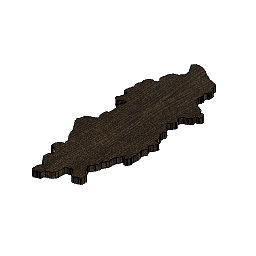
model (Autodesk Fusion 360 design; units mm, degrees)
Autodesk Fusion 360 part; units mm, degrees
(part 1 of 2)
sketch "Sketch1" plane through (0, 0, 0) normal (0, 0, 1) x (1, 0, 0)
  spline S0 degree 3 poles (85.9896, 120.8052) (84.9842, 121.2285) (83.9523, 120.9375) (82.9998, 120.8052) knots 0 0 0 0 1 1 1 1
  spline S1 degree 3 poles (82.9998, 120.8052) (82.0738, 120.6994) (81.4123, 120.911) (80.8038, 121.4667) knots 0 0 0 0 1 1 1 1
  spline S2 degree 3 poles (80.8038, 121.4667) (80.645, 121.6254) (80.4863, 121.89) (80.4863, 122.1017) knots 0 0 0 0 1 1 1 1
  spline S3 degree 3 poles (80.4863, 122.1017) (80.5127, 122.7102) (80.5921, 123.3187) (80.645, 123.9273) knots 0 0 0 0 1 1 1 1
  spline S4 degree 3 poles (80.645, 123.9273) (80.645, 123.9802) (80.6715, 124.0331) (80.6979, 124.086) knots 0 0 0 0 1 1 1 1
  spline S5 degree 3 poles (80.6979, 124.086) (80.989, 124.6681) (81.1742, 125.356) (79.9042, 127.605) knots 0 0 0 0 1 1 1 1
  spline S6 degree 2 poles (79.9042, 127.605) (79.9042, 127.6315) (79.8777, 127.6579) knots 0 0 0 1 1 1
  spline S7 degree 3 poles (79.8777, 127.6579) (79.7719, 127.9225) (79.6925, 128.1606) (79.5867, 128.4252) knots 0 0 0 0 1 1 1 1
  spline S8 degree 3 poles (79.5867, 128.4252) (79.0575, 129.6158) (78.6077, 130.8594) (77.4435, 131.6796) knots 0 0 0 0 1 1 1 1
  spline S9 degree 3 poles (77.4435, 131.6796) (77.0731, 131.9442) (76.835, 132.4998) (76.7556, 132.976) knots 0 0 0 0 1 1 1 1
  spline S10 degree 3 poles (76.7556, 132.976) (76.6763, 133.4523) (76.8615, 133.9814) (76.9408, 134.4577) knots 0 0 0 0 1 1 1 1
  spline S11 degree 3 poles (76.9408, 134.4577) (77.0996, 135.516) (77.1525, 136.6008) (77.6817, 137.5798) knots 0 0 0 0 1 1 1 1
  spline S12 degree 3 poles (77.6817, 137.5798) (78.105, 138.3735) (77.8669, 139.3789) (77.0996, 139.8817) knots 0 0 0 0 1 1 1 1
  spline S13 degree 3 poles (77.0996, 139.8817) (76.6498, 140.1992) (76.4381, 140.596) (76.4381, 141.1781) knots 0 0 0 0 1 1 1 1
  spline S14 degree 3 poles (76.4381, 141.1781) (76.4381, 141.6544) (76.2529, 141.9983) (75.7502, 142.21) knots 0 0 0 0 1 1 1 1
  spline S15 degree 3 poles (75.7502, 142.21) (75.0887, 142.4746) (74.5596, 142.9508) (74.2156, 143.6123) knots 0 0 0 0 1 1 1 1
  spline S16 degree 3 poles (74.2156, 143.6123) (74.0833, 143.8769) (73.7658, 144.0621) (73.5012, 144.2208) knots 0 0 0 0 1 1 1 1
  spline S17 degree 3 poles (73.5012, 144.2208) (72.3371, 144.9352) (70.9612, 145.3585) (70.3792, 146.7608) knots 0 0 0 0 1 1 1 1
  spline S18 degree 3 poles (70.3792, 146.7608) (70.141, 147.3429) (69.9029, 147.925) (69.7177, 148.5071) knots 0 0 0 0 1 1 1 1
  spline S19 degree 3 poles (69.7177, 148.5071) (69.215, 149.9623) (69.506, 150.9148) (70.7231, 151.8673) knots 0 0 0 0 1 1 1 1
  spline S20 degree 3 poles (70.7231, 151.8673) (71.3581, 152.37) (72.046, 152.8198) (72.1519, 153.7194) knots 0 0 0 0 1 1 1 1
  spline S21 degree 3 poles (72.1519, 153.7194) (72.2577, 154.6719) (72.7604, 155.4656) (73.369, 156.2064) knots 0 0 0 0 1 1 1 1
  spline S22 degree 3 poles (73.369, 156.2064) (73.5277, 156.4181) (73.6865, 156.6298) (73.7923, 156.8679) knots 0 0 0 0 1 1 1 1
  spline S23 degree 3 poles (73.7923, 156.8679) (73.8717, 157.0002) (73.951, 157.1854) (73.8981, 157.3177) knots 0 0 0 0 1 1 1 1
  spline S24 degree 3 poles (73.8981, 157.3177) (73.5806, 158.5348) (73.4748, 159.8312) (72.3106, 160.6779) knots 0 0 0 0 1 1 1 1
  spline S25 degree 3 poles (72.3106, 160.6779) (71.3317, 161.3923) (70.5644, 162.2919) (70.2469, 163.5354) knots 0 0 0 0 1 1 1 1
  spline S26 degree 3 poles (70.2469, 163.5354) (70.194, 163.7206) (70.141, 163.9323) (70.1675, 164.1175) knots 0 0 0 0 1 1 1 1
  spline S27 degree 3 poles (70.1675, 164.1175) (70.4056, 165.6785) (71.2523, 166.9221) (72.6017, 167.6894) knots 0 0 0 0 1 1 1 1
  spline S28 degree 3 poles (72.6017, 167.6894) (73.8981, 168.4302) (75.274, 169.0387) (76.5969, 169.7531) knots 0 0 0 0 1 1 1 1
  spline S29 degree 3 poles (76.5969, 169.7531) (76.8879, 169.9119) (77.2054, 170.1235) (77.3377, 170.3881) knots 0 0 0 0 1 1 1 1
  spline S30 degree 3 poles (77.3377, 170.3881) (77.6552, 171.1289) (78.1579, 171.6581) (78.8458, 172.0814) knots 0 0 0 0 1 1 1 1
  spline S31 degree 3 poles (78.8458, 172.0814) (79.3221, 172.3725) (79.9835, 172.6635) (80.1688, 173.1133) knots 0 0 0 0 1 1 1 1
  spline S32 degree 3 poles (80.1688, 173.1133) (80.5127, 173.9071) (80.8831, 174.8067) (80.1423, 175.6533) knots 0 0 0 0 1 1 1 1
  spline S33 degree 3 poles (80.1423, 175.6533) (79.4015, 176.5) (79.9306, 177.0556) (80.8302, 177.2937) knots 0 0 0 0 1 1 1 1
  spline S34 degree 3 poles (80.8302, 177.2937) (81.5181, 177.4789) (82.2325, 177.5583) (82.894, 177.7964) knots 0 0 0 0 1 1 1 1
  spline S35 degree 3 poles (82.894, 177.7964) (83.3967, 177.9817) (84.0052, 178.2198) (84.2169, 178.6431) knots 0 0 0 0 1 1 1 1
  spline S36 degree 3 poles (84.2169, 178.6431) (84.6667, 179.5162) (84.9842, 180.4687) (85.1958, 181.4477) knots 0 0 0 0 1 1 1 1
  spline S37 degree 3 poles (85.1958, 181.4477) (85.3017, 182.0033) (85.2223, 182.6912) (84.9577, 183.1939) knots 0 0 0 0 1 1 1 1
  spline S38 degree 3 poles (84.9577, 183.1939) (84.6931, 183.7231) (84.164, 184.12) (83.6877, 184.4904) knots 0 0 0 0 1 1 1 1
  spline S39 degree 3 poles (83.6877, 184.4904) (83.2644, 184.8079) (82.7617, 185.046) (82.259, 185.2312) knots 0 0 0 0 1 1 1 1
  spline S40 degree 3 poles (82.259, 185.2312) (81.1742, 185.6017) (80.1423, 185.1519) (79.084, 184.9667) knots 0 0 0 0 1 1 1 1
  spline S41 degree 3 poles (79.084, 184.9667) (78.8988, 184.9402) (78.6606, 184.8608) (78.5019, 184.9402) knots 0 0 0 0 1 1 1 1
  spline S42 degree 3 poles (78.5019, 184.9402) (78.2108, 185.0196) (77.814, 185.5752) (77.5758, 186.0779) knots 0 0 0 0 1 1 1 1
  spline S43 degree 3 poles (77.5758, 186.0779) (77.5494, 186.1308) (77.5494, 186.1573) (77.5229, 186.2102) knots 0 0 0 0 1 1 1 1
  spline S44 degree 3 poles (77.5229, 186.2102) (77.47, 186.4483) (77.4171, 186.66) (77.3377, 186.8452) knots 0 0 0 0 1 1 1 1
  spline S45 degree 3 poles (77.3377, 186.8452) (75.7502, 190.0996) (73.9246, 188.4856) (67.7598, 191.7135) knots 0 0 0 0 1 1 1 1
  spline S46 degree 3 poles (67.7598, 191.7135) (64.77, 193.2746) (62.7856, 195.5235) (61.5421, 197.4285) knots 0 0 0 0 1 1 1 1
  spline S47 degree 3 poles (61.5421, 197.4285) (61.5156, 197.455) (61.5156, 197.4814) (61.4892, 197.5344) knots 0 0 0 0 1 1 1 1
  spline S48 degree 3 poles (61.4892, 197.5344) (61.4098, 197.746) (61.3304, 197.9312) (61.251, 198.1429) knots 0 0 0 0 1 1 1 1
  spline S49 degree 3 poles (61.251, 198.1429) (61.1717, 198.3017) (61.1188, 198.4604) (60.9865, 198.5133) knots 0 0 0 0 1 1 1 1
  spline S50 degree 3 poles (60.9865, 198.5133) (60.9071, 198.5662) (60.8013, 198.6191) (60.7483, 198.725) knots 0 0 0 0 1 1 1 1
  spline S51 degree 2 poles (60.7483, 198.725) (60.0075, 200.1008) (59.7165, 201.0533) knots 0 0 0 1 1 1
  line L0 (59.7165, 201.0533) -> (59.69, 201.2385)
  spline S52 degree 3 poles (59.69, 201.2385) (59.6106, 202.0852) (60.0869, 202.6408) (60.6954, 203.1964) knots 0 0 0 0 1 1 1 1
  spline S53 degree 3 poles (60.6954, 203.1964) (60.8277, 203.3287) (60.8806, 203.6462) (60.8542, 203.8844) knots 0 0 0 0 1 1 1 1
  spline S54 degree 3 poles (60.8542, 203.8844) (60.8013, 204.3871) (60.5102, 204.7046) (60.034, 204.9162) knots 0 0 0 0 1 1 1 1
  spline S55 degree 3 poles (60.034, 204.9162) (59.9546, 204.9427) (59.8752, 204.9956) (59.7958, 205.0485) knots 0 0 0 0 1 1 1 1
  spline S56 degree 3 poles (59.7958, 205.0485) (59.5313, 205.2073) (59.4783, 205.5777) (59.69, 205.8158) knots 0 0 0 0 1 1 1 1
  spline S57 degree 3 poles (59.69, 205.8158) (59.9546, 206.1069) (60.1927, 206.2391) (60.5631, 206.2656) knots 0 0 0 0 1 1 1 1
  spline S58 degree 3 poles (60.5631, 206.2656) (60.8806, 206.2921) (61.0923, 206.636) (60.96, 206.9271) knots 0 0 0 0 1 1 1 1
  spline S59 degree 3 poles (60.96, 206.9271) (60.6161, 207.7473) (60.0604, 208.4087) (59.5048, 209.0966) knots 0 0 0 0 1 1 1 1
  spline S60 degree 3 poles (59.5048, 209.0966) (58.3936, 210.4989) (58.6846, 212.2981) (60.1927, 213.0919) knots 0 0 0 0 1 1 1 1
  spline S61 degree 3 poles (60.1927, 213.0919) (60.6161, 213.3035) (61.1188, 213.33) (61.6479, 213.3829) knots 0 0 0 0 1 1 1 1
  spline S62 degree 3 poles (61.6479, 213.3829) (61.939, 213.4094) (62.1771, 213.7004) (62.0977, 213.9914) knots 0 0 0 0 1 1 1 1
  spline S63 degree 3 poles (62.0977, 213.9914) (61.939, 214.5206) (61.7273, 215.0762) (61.5421, 215.6054) knots 0 0 0 0 1 1 1 1
  spline S64 degree 3 poles (61.5421, 215.6054) (61.5421, 215.6319) (61.5156, 215.6583) (61.5156, 215.6848) knots 0 0 0 0 1 1 1 1
  spline S65 degree 3 poles (61.5156, 215.6848) (61.1717, 216.2669) (61.0923, 216.9019) (61.2246, 217.5898) knots 0 0 0 0 1 1 1 1
  spline S66 degree 3 poles (61.2246, 217.5898) (61.3569, 218.2512) (61.3569, 218.9127) (61.3833, 219.5741) knots 0 0 0 0 1 1 1 1
  spline S67 degree 3 poles (61.3833, 219.5741) (61.4098, 220.1033) (61.0923, 220.3944) (60.6425, 220.5266) knots 0 0 0 0 1 1 1 1
  spline S68 degree 3 poles (60.6425, 220.5266) (60.4044, 220.606) (60.1398, 220.6589) (59.8752, 220.7119) knots 0 0 0 0 1 1 1 1
  spline S69 degree 3 poles (59.8752, 220.7119) (58.7904, 220.95) (58.129, 221.9554) (58.1819, 223.0402) knots 0 0 0 0 1 1 1 1
  spline S70 degree 3 poles (58.1819, 223.0402) (58.2083, 223.5164) (58.0496, 223.8869) (57.6527, 224.2308) knots 0 0 0 0 1 1 1 1
  spline S71 degree 3 poles (57.6527, 224.2308) (56.8325, 224.9981) (56.6473, 226.03) (57.1236, 227.0619) knots 0 0 0 0 1 1 1 1
  spline S72 degree 3 poles (57.1236, 227.0619) (57.1765, 227.1677) (57.2029, 227.3264) (57.15, 227.3794) knots 0 0 0 0 1 1 1 1
  spline S73 degree 3 poles (57.15, 227.3794) (56.8061, 227.8821) (56.6208, 228.57) (55.8271, 228.6758) knots 0 0 0 0 1 1 1 1
  spline S74 degree 3 poles (55.8271, 228.6758) (44.9792, 230.2369) (37.2798, 234.3908) (34.2371, 236.5604) knots 0 0 0 0 1 1 1 1
  spline S75 degree 3 poles (34.2371, 236.5604) (34.2106, 236.5604) (34.2106, 236.5869) (34.1842, 236.5869) knots 0 0 0 0 1 1 1 1
  spline S76 degree 3 poles (34.1842, 236.5869) (34.1313, 236.6398) (34.0783, 236.6927) (34.0254, 236.7456) knots 0 0 0 0 1 1 1 1
  spline S77 degree 3 poles (34.0254, 236.7456) (33.999, 236.7721) (33.9725, 236.7985) (33.946, 236.7985) knots 0 0 0 0 1 1 1 1
  spline S78 degree 3 poles (33.946, 236.7985) (33.8931, 236.825) (33.8402, 236.8779) (33.7608, 236.9044) knots 0 0 0 0 1 1 1 1
  spline S79 degree 3 poles (33.7608, 236.9044) (33.7344, 236.9044) (33.7344, 236.9308) (33.7079, 236.9308) knots 0 0 0 0 1 1 1 1
  spline S80 degree 3 poles (33.7079, 236.9308) (31.1679, 238.8623) (26.5906, 239.7619) (26.1144, 239.8413) knots 0 0 0 0 1 1 1 1
  spline S81 degree 3 poles (26.1144, 239.8413) (26.0879, 239.8413) (26.0615, 239.8413) (26.035, 239.8413) knots 0 0 0 0 1 1 1 1
  spline S82 degree 3 poles (26.035, 239.8413) (25.0296, 239.8942) (24.0242, 239.9206) (23.0188, 239.9735) knots 0 0 0 0 1 1 1 1
  spline S83 degree 3 poles (23.0188, 239.9735) (22.8865, 239.9735) (22.7542, 240) (22.6219, 240) knots 0 0 0 0 1 1 1 1
  spline S84 degree 3 poles (22.6219, 240) (22.569, 240) (22.5425, 240) (22.4896, 240) knots 0 0 0 0 1 1 1 1
  spline S85 degree 3 poles (22.4896, 240) (21.5371, 239.8148) (20.5846, 239.656) (19.6321, 239.4708) knots 0 0 0 0 1 1 1 1
  spline S86 degree 3 poles (19.6321, 239.4708) (19.5792, 239.4444) (19.4998, 239.4179) (19.4469, 239.3915) knots 0 0 0 0 1 1 1 1
  spline S87 degree 3 poles (19.4469, 239.3915) (19.394, 239.365) (19.3675, 239.3385) (19.341, 239.3121) knots 0 0 0 0 1 1 1 1
  line L1 (19.341, 239.3121) -> (19.2087, 239.1798)
  spline S88 degree 3 poles (19.2087, 239.1798) (19.1823, 239.1533) (19.1558, 239.1269) (19.1029, 239.1004) knots 0 0 0 0 1 1 1 1
  spline S89 degree 3 poles (19.1029, 239.1004) (18.7854, 238.9417) (18.4944, 238.8094) (18.2033, 238.6506) knots 0 0 0 0 1 1 1 1
  line L2 (18.2033, 238.6506) -> (18.0446, 238.5448)
  spline S90 degree 3 poles (18.0446, 238.5448) (17.9917, 238.4919) (17.9388, 238.439) (17.8858, 238.3596) knots 0 0 0 0 1 1 1 1
  spline S91 degree 3 poles (17.8858, 238.3596) (17.8594, 238.3331) (17.8594, 238.2802) (17.8329, 238.2538) knots 0 0 0 0 1 1 1 1
  spline S92 degree 3 poles (17.8329, 238.2538) (16.9333, 237.5658) (16.2719, 236.7192) (15.875, 235.6608) knots 0 0 0 0 1 1 1 1
  spline S93 degree 3 poles (15.875, 235.6608) (15.8221, 235.5285) (15.8485, 235.3698) (15.9279, 235.2375) knots 0 0 0 0 1 1 1 1
  spline S94 degree 3 poles (15.9279, 235.2375) (16.0073, 235.1052) (16.1131, 234.9465) (16.1925, 234.8142) knots 0 0 0 0 1 1 1 1
  spline S95 degree 3 poles (16.1925, 234.8142) (16.4306, 234.4967) (16.6688, 234.1792) (16.9333, 233.8352) knots 0 0 0 0 1 1 1 1
  spline S96 degree 3 poles (16.9333, 233.8352) (18.6002, 231.4275) (20.2406, 228.9669) (21.934, 226.5856) knots 0 0 0 0 1 1 1 1
  spline S97 degree 3 poles (21.934, 226.5856) (22.4102, 225.9242) (22.516, 225.2098) (22.6483, 224.4954) knots 0 0 0 0 1 1 1 1
  spline S98 degree 3 poles (22.6483, 224.4954) (22.8335, 223.3312) (22.9923, 222.1671) (23.151, 221.0029) knots 0 0 0 0 1 1 1 1
  spline S99 degree 3 poles (23.151, 221.0029) (23.204, 220.606) (23.1246, 220.2092) (22.9129, 219.8652) knots 0 0 0 0 1 1 1 1
  spline S100 degree 3 poles (22.9129, 219.8652) (22.5954, 219.3096) (22.2515, 218.7804) (21.881, 218.2512) knots 0 0 0 0 1 1 1 1
  spline S101 degree 3 poles (21.881, 218.2512) (21.7488, 218.066) (21.5635, 217.8808) (21.3519, 217.775) knots 0 0 0 0 1 1 1 1
  spline S102 degree 3 poles (21.3519, 217.775) (20.664, 217.4575) (20.3465, 216.8754) (20.1083, 216.214) knots 0 0 0 0 1 1 1 1
  spline S103 degree 3 poles (20.1083, 216.214) (19.8967, 215.579) (19.5263, 215.1027) (18.8648, 214.8117) knots 0 0 0 0 1 1 1 1
  spline S104 degree 3 poles (18.8648, 214.8117) (17.3302, 214.0973) (15.7956, 213.33) (14.2875, 212.5362) knots 0 0 0 0 1 1 1 1
  spline S105 degree 3 poles (14.2875, 212.5362) (13.1763, 211.9277) (12.5148, 210.8429) (12.0915, 209.7052) knots 0 0 0 0 1 1 1 1
  spline S106 degree 3 poles (12.0915, 209.7052) (11.6417, 208.4881) (11.4565, 207.1917) (11.0331, 205.9746) knots 0 0 0 0 1 1 1 1
  spline S107 degree 3 poles (11.0331, 205.9746) (11.0067, 205.8687) (10.9538, 205.7894) (10.9273, 205.6835) knots 0 0 0 0 1 1 1 1
  spline S108 degree 3 poles (10.9273, 205.6835) (10.9008, 205.6042) (10.9008, 205.5512) (10.9008, 205.4719) knots 0 0 0 0 1 1 1 1
  spline S109 degree 3 poles (10.9008, 205.4719) (10.9008, 205.3131) (10.9273, 205.1544) (10.9273, 204.9692) knots 0 0 0 0 1 1 1 1
  spline S110 degree 3 poles (10.9273, 204.9692) (10.9273, 204.1225) (10.7685, 203.3287) (10.451, 202.6144) knots 0 0 0 0 1 1 1 1
  spline S111 degree 3 poles (10.451, 202.6144) (10.4246, 202.5879) (10.4246, 202.535) (10.4246, 202.5085) knots 0 0 0 0 1 1 1 1
  spline S112 degree 3 poles (10.4246, 202.5085) (10.3188, 201.8735) (10.2129, 201.3444) (10.16, 200.7888) knots 0 0 0 0 1 1 1 1
  spline S113 degree 3 poles (10.16, 200.7888) (10.0013, 199.5717) (9.9483, 198.381) (10.7421, 197.3492) knots 0 0 0 0 1 1 1 1
  spline S114 degree 3 poles (10.7421, 197.3492) (11.2448, 196.6877) (11.8798, 196.1321) (12.3825, 195.4971) knots 0 0 0 0 1 1 1 1
  spline S115 degree 3 poles (12.3825, 195.4971) (12.5942, 195.2325) (12.7794, 194.8621) (12.7529, 194.5446) knots 0 0 0 0 1 1 1 1
  spline S116 degree 3 poles (12.7529, 194.5446) (12.7265, 193.8831) (12.6735, 193.2481) (12.5677, 192.5867) knots 0 0 0 0 1 1 1 1
  spline S117 degree 3 poles (12.5677, 192.5867) (12.5148, 192.1633) (11.9856, 192.0046) (11.721, 192.2956) knots 0 0 0 0 1 1 1 1
  spline S118 degree 3 poles (11.721, 192.2956) (11.5623, 192.4808) (11.3771, 192.6396) (11.1125, 192.719) knots 0 0 0 0 1 1 1 1
  spline S119 degree 3 poles (11.1125, 192.719) (10.9008, 192.7983) (10.6627, 192.719) (10.5569, 192.5338) knots 0 0 0 0 1 1 1 1
  spline S120 degree 3 poles (10.5569, 192.5338) (10.3188, 192.1898) (10.1865, 191.7929) (10.1071, 191.3696) knots 0 0 0 0 1 1 1 1
  spline S121 degree 3 poles (10.1071, 191.3696) (10.0277, 191.0256) (9.6044, 190.8669) (9.3133, 191.0785) knots 0 0 0 0 1 1 1 1
  spline S122 degree 3 poles (9.3133, 191.0785) (9.1281, 191.2373) (8.9165, 191.3696) (8.6783, 191.4754) knots 0 0 0 0 1 1 1 1
  spline S123 degree 3 poles (8.6783, 191.4754) (8.3873, 191.6077) (7.8846, 191.6871) (7.5671, 191.6077) knots 0 0 0 0 1 1 1 1
  spline S124 degree 3 poles (7.5671, 191.6077) (5.7679, 191.1579) (4.3392, 190.126) (2.9898, 188.909) knots 0 0 0 0 1 1 1 1
  spline S125 degree 3 poles (2.9898, 188.909) (2.8046, 188.7502) (2.7252, 188.4592) (2.6988, 188.221) knots 0 0 0 0 1 1 1 1
  spline S126 degree 3 poles (2.6988, 188.221) (2.5929, 187.5331) (2.4871, 186.8717) (1.9844, 186.316) knots 0 0 0 0 1 1 1 1
  spline S127 degree 3 poles (1.9844, 186.316) (1.4023, 185.681) (1.4817, 184.9138) (1.4552, 184.12) knots 0 0 0 0 1 1 1 1
  spline S128 degree 3 poles (1.4552, 184.12) (1.4288, 183.2998) (1.4817, 182.5854) (2.2754, 182.1092) knots 0 0 0 0 1 1 1 1
  spline S129 degree 3 poles (2.2754, 182.1092) (2.3283, 182.0827) (2.4342, 181.9769) (2.4342, 181.924) knots 0 0 0 0 1 1 1 1
  spline S130 degree 3 poles (2.4342, 181.924) (2.3813, 181.1302) (2.5665, 180.2306) (1.9579, 179.5956) knots 0 0 0 0 1 1 1 1
  spline S131 degree 3 poles (1.9579, 179.5956) (1.0583, 178.6431) (0.6085, 177.6112) (0.7144, 176.3148) knots 0 0 0 0 1 1 1 1
  spline S132 degree 3 poles (0.7144, 176.3148) (0.7938, 175.4946) (0.7144, 174.6744) (0.7408, 173.8542) knots 0 0 0 0 1 1 1 1
  spline S133 degree 3 poles (0.7408, 173.8542) (0.7408, 173.5367) (0.979, 173.1133) (1.2435, 172.9017) knots 0 0 0 0 1 1 1 1
  spline S134 degree 3 poles (1.2435, 172.9017) (1.9844, 172.346) (2.1696, 171.4729) (2.1431, 170.7056) knots 0 0 0 0 1 1 1 1
  spline S135 degree 3 poles (2.1431, 170.7056) (2.0638, 168.9065) (1.4817, 167.1867) (0.8731, 165.4669) knots 0 0 0 0 1 1 1 1
  spline S136 degree 3 poles (0.8731, 165.4669) (0.4498, 164.2498) (0.3969, 162.9269) (0.1058, 161.6569) knots 0 0 0 0 1 1 1 1
  spline S137 degree 3 poles (0.1058, 161.6569) (-0.0794, 160.8102) (0.1588, 160.0165) (0.5821, 159.4608) knots 0 0 0 0 1 1 1 1
  spline S138 degree 3 poles (0.5821, 159.4608) (1.1906, 158.6936) (2.0373, 158.0321) (3.0956, 157.9263) knots 0 0 0 0 1 1 1 1
  spline S139 degree 3 poles (3.0956, 157.9263) (3.3073, 157.8998) (3.5454, 158.1379) (3.7306, 158.2967) knots 0 0 0 0 1 1 1 1
  spline S140 degree 3 poles (3.7306, 158.2967) (4.2598, 158.7729) (4.6038, 158.6936) (4.8154, 158.0056) knots 0 0 0 0 1 1 1 1
  spline S141 degree 3 poles (4.8154, 158.0056) (5.2123, 156.7356) (5.3181, 155.4392) (5.0271, 154.1163) knots 0 0 0 0 1 1 1 1
  spline S142 degree 3 poles (5.0271, 154.1163) (4.9213, 153.6135) (4.9477, 153.0579) (4.8683, 152.5552) knots 0 0 0 0 1 1 1 1
  spline S143 degree 3 poles (4.8683, 152.5552) (4.8419, 152.2906) (4.7096, 152.026) (4.6302, 151.7615) knots 0 0 0 0 1 1 1 1
  spline S144 degree 3 poles (4.6302, 151.7615) (4.5773, 151.7085) (4.5508, 151.6292) (4.4979, 151.5763) knots 0 0 0 0 1 1 1 1
  spline S145 degree 3 poles (4.4979, 151.5763) (4.0746, 150.2004) (3.2808, 149.0363) (2.4077, 147.8985) knots 0 0 0 0 1 1 1 1
  spline S146 degree 3 poles (2.4077, 147.8985) (2.0108, 147.3958) (1.905, 146.7873) (2.1431, 146.0994) knots 0 0 0 0 1 1 1 1
  spline S147 degree 3 poles (2.1431, 146.0994) (2.7517, 144.3796) (4.2069, 143.6388) (5.6885, 142.9244) knots 0 0 0 0 1 1 1 1
  spline S148 degree 3 poles (5.6885, 142.9244) (6.006, 142.7656) (6.3235, 142.6863) (6.641, 142.554) knots 0 0 0 0 1 1 1 1
  spline S149 degree 3 poles (6.641, 142.554) (7.2496, 142.2894) (7.9375, 142.3952) (8.2021, 142.9773) knots 0 0 0 0 1 1 1 1
  spline S150 degree 3 poles (8.2021, 142.9773) (8.8635, 144.4325) (10.2129, 145.1204) (11.2977, 146.0994) knots 0 0 0 0 1 1 1 1
  spline S151 degree 3 poles (11.2977, 146.0994) (11.8269, 146.6021) (12.3825, 147.0783) (12.8852, 147.6075) knots 0 0 0 0 1 1 1 1
  spline S152 degree 3 poles (12.8852, 147.6075) (13.4673, 148.2425) (14.0229, 147.6869) (14.5785, 147.634) knots 0 0 0 0 1 1 1 1
  spline S153 degree 3 poles (14.5785, 147.634) (15.0019, 147.6075) (14.9225, 147.2106) (15.0019, 146.9461) knots 0 0 0 0 1 1 1 1
  spline S154 degree 3 poles (15.0019, 146.9461) (15.5046, 145.5438) (14.6579, 144.4061) (14.2346, 143.2154) knots 0 0 0 0 1 1 1 1
  spline S155 degree 3 poles (14.2346, 143.2154) (14.2346, 143.189) (14.2346, 143.189) (14.2081, 143.1625) knots 0 0 0 0 1 1 1 1
  spline S156 degree 3 poles (14.2081, 143.1625) (14.0229, 142.8186) (13.8642, 142.4481) (13.7054, 142.0777) knots 0 0 0 0 1 1 1 1
  spline S157 degree 2 poles (13.7054, 142.0777) (13.7054, 142.0513) (13.679, 142.0513) knots 0 0 0 1 1 1
  spline S158 degree 3 poles (13.679, 142.0513) (13.5467, 141.7867) (13.3879, 141.5221) (13.2556, 141.231) knots 0 0 0 0 1 1 1 1
  spline S159 degree 3 poles (13.2556, 141.231) (13.2821, 141.231) (13.335, 141.231) (13.3615, 141.231) knots 0 0 0 0 1 1 1 1
  spline S160 degree 3 poles (13.3615, 141.231) (12.8058, 139.7758) (12.3825, 138.3471) (12.2502, 137.7915) knots 0 0 0 0 1 1 1 1
  spline S161 degree 3 poles (12.2502, 137.7915) (12.2238, 137.7121) (12.1973, 137.6327) (12.1708, 137.5269) knots 0 0 0 0 1 1 1 1
  spline S162 degree 3 poles (12.1708, 137.5269) (12.1179, 137.2888) (12.0385, 137.0506) (12.065, 136.8125) knots 0 0 0 0 1 1 1 1
  spline S163 degree 3 poles (12.065, 136.8125) (12.0915, 136.5744) (12.1708, 136.2833) (12.356, 136.1775) knots 0 0 0 0 1 1 1 1
  spline S164 degree 3 poles (12.356, 136.1775) (12.8852, 135.7806) (13.4408, 135.4102) (14.0494, 135.1192) knots 0 0 0 0 1 1 1 1
  spline S165 degree 3 poles (14.0494, 135.1192) (15.1342, 134.59) (15.4517, 133.611) (15.531, 132.5792) knots 0 0 0 0 1 1 1 1
  spline S166 degree 3 poles (15.531, 132.5792) (15.6104, 131.2298) (15.4781, 129.8275) (15.4781, 128.4781) knots 0 0 0 0 1 1 1 1
  spline S167 degree 3 poles (15.4781, 128.4781) (15.4781, 128.1077) (15.584, 127.7637) (15.5575, 127.3933) knots 0 0 0 0 1 1 1 1
  spline S168 degree 3 poles (15.5575, 127.3933) (15.5046, 125.8852) (15.4252, 124.4035) (15.2929, 122.8954) knots 0 0 0 0 1 1 1 1
  spline S169 degree 3 poles (15.2929, 122.8954) (15.2929, 122.7367) (14.9754, 122.4985) (14.7902, 122.4456) knots 0 0 0 0 1 1 1 1
  spline S170 degree 3 poles (14.7902, 122.4456) (14.4463, 122.3662) (14.0494, 122.3927) (13.7054, 122.4192) knots 0 0 0 0 1 1 1 1
  spline S171 degree 3 poles (13.7054, 122.4192) (13.2821, 122.4456) (13.0704, 122.2869) (12.9381, 121.9165) knots 0 0 0 0 1 1 1 1
  spline S172 degree 3 poles (12.9381, 121.9165) (12.2502, 120.0379) (12.0915, 118.1329) (12.8588, 116.2279) knots 0 0 0 0 1 1 1 1
  spline S173 degree 3 poles (12.8588, 116.2279) (12.9381, 116.0427) (12.9381, 115.8046) (12.9381, 115.5929) knots 0 0 0 0 1 1 1 1
  spline S174 degree 3 poles (12.9381, 115.5929) (12.8058, 114.2435) (12.8058, 112.9735) (13.97, 111.9681) knots 0 0 0 0 1 1 1 1
  spline S175 degree 3 poles (13.97, 111.9681) (14.8431, 111.2273) (15.0813, 109.6927) (14.4198, 108.7667) knots 0 0 0 0 1 1 1 1
  spline S176 degree 3 poles (14.4198, 108.7667) (14.3669, 108.6873) (14.3404, 108.555) (14.261, 108.5021) knots 0 0 0 0 1 1 1 1
  spline S177 degree 3 poles (14.261, 108.5021) (13.4938, 108.0787) (12.7, 107.6819) (11.9063, 107.2585) knots 0 0 0 0 1 1 1 1
  spline S178 degree 3 poles (11.9063, 107.2585) (11.8533, 107.2056) (11.8269, 107.1527) (11.774, 107.1262) knots 0 0 0 0 1 1 1 1
  spline S179 degree 3 poles (11.774, 107.1262) (11.0331, 106.6764) (10.3188, 106.1737) (9.5779, 105.7504) knots 0 0 0 0 1 1 1 1
  spline S180 degree 3 poles (9.5779, 105.7504) (8.6519, 105.2477) (7.6465, 104.8508) (6.694, 104.4275) knots 0 0 0 0 1 1 1 1
  line L3 (6.694, 104.4275) -> (6.4558, 104.2423)
  spline S181 degree 3 poles (6.4558, 104.2423) (5.7944, 103.4485) (5.1065, 102.6283) (4.445, 101.8346) knots 0 0 0 0 1 1 1 1
  spline S182 degree 3 poles (4.445, 101.8346) (4.3656, 101.7287) (4.2598, 101.5964) (4.1275, 101.57) knots 0 0 0 0 1 1 1 1
  spline S183 degree 3 poles (4.1275, 101.57) (3.2279, 101.226) (3.175, 100.4587) (3.0956, 99.6385) knots 0 0 0 0 1 1 1 1
  spline S184 degree 3 poles (3.0956, 99.6385) (2.9898, 98.6067) (2.884, 97.5219) (2.5929, 96.5429) knots 0 0 0 0 1 1 1 1
  spline S185 degree 3 poles (2.5929, 96.5429) (2.3548, 95.7227) (1.8256, 94.9819) (1.4552, 94.2146) knots 0 0 0 0 1 1 1 1
  spline S186 degree 3 poles (1.4552, 94.2146) (1.3229, 93.95) (1.2435, 93.606) (1.27, 93.315) knots 0 0 0 0 1 1 1 1
  spline S187 degree 3 poles (1.27, 93.315) (1.4288, 91.4629) (2.3283, 89.9548) (3.519, 88.5789) knots 0 0 0 0 1 1 1 1
  spline S188 degree 3 poles (3.519, 88.5789) (4.1275, 87.891) (4.6302, 87.1237) (5.2652, 86.4623) knots 0 0 0 0 1 1 1 1
  spline S189 degree 3 poles (5.2652, 86.4623) (7.1967, 84.4779) (8.3344, 81.9379) (10.2394, 79.9535) knots 0 0 0 0 1 1 1 1
  spline S190 degree 3 poles (10.2394, 79.9535) (10.4775, 79.7154) (10.6627, 79.4244) (10.9273, 79.2656) knots 0 0 0 0 1 1 1 1
  spline S191 degree 3 poles (10.9273, 79.2656) (11.6417, 78.7894) (11.8533, 78.075) (11.9856, 77.3077) knots 0 0 0 0 1 1 1 1
  spline S192 degree 3 poles (11.9856, 77.3077) (12.2502, 75.6937) (12.7265, 74.1592) (13.5467, 72.7304) knots 0 0 0 0 1 1 1 1
  spline S193 degree 3 poles (13.5467, 72.7304) (14.5521, 70.9312) (15.4517, 69.0527) (16.5365, 67.3065) knots 0 0 0 0 1 1 1 1
  spline S194 degree 3 poles (16.5365, 67.3065) (17.2773, 66.1158) (18.2298, 65.0839) (19.1294, 63.9992) knots 0 0 0 0 1 1 1 1
  spline S195 degree 3 poles (19.1294, 63.9992) (19.7644, 63.2054) (20.4258, 62.4381) (21.0608, 61.6444) knots 0 0 0 0 1 1 1 1
  spline S196 degree 3 poles (21.0608, 61.6444) (21.1931, 61.4592) (21.299, 61.1681) (21.246, 60.9829) knots 0 0 0 0 1 1 1 1
  spline S197 degree 3 poles (21.246, 60.9829) (20.955, 59.5277) (21.2196, 58.0989) (21.5635, 56.6967) knots 0 0 0 0 1 1 1 1
  spline S198 degree 3 poles (21.5635, 56.6967) (21.6958, 56.0881) (21.5371, 55.9029) (21.0079, 55.7971) knots 0 0 0 0 1 1 1 1
  spline S199 degree 3 poles (21.0079, 55.7971) (19.6321, 55.4796) (18.4679, 54.6329) (17.4625, 53.7333) knots 0 0 0 0 1 1 1 1
  spline S200 degree 3 poles (17.4625, 53.7333) (16.5894, 52.9396) (15.875, 51.8812) (15.5046, 50.6377) knots 0 0 0 0 1 1 1 1
  spline S201 degree 3 poles (15.5046, 50.6377) (15.1606, 49.3941) (14.8167, 48.1771) (14.949, 46.8806) knots 0 0 0 0 1 1 1 1
  line L4 (14.949, 46.8806) -> (14.949, 46.8542)
  spline S202 degree 3 poles (14.949, 46.8542) (14.949, 46.7483) (14.949, 46.6689) (14.949, 46.5631) knots 0 0 0 0 1 1 1 1
  spline S203 degree 3 poles (14.949, 46.5631) (14.949, 46.5367) (14.949, 46.4837) (14.949, 46.4573) knots 0 0 0 0 1 1 1 1
  spline S204 degree 3 poles (14.949, 46.4573) (15.0019, 46.1398) (15.0548, 45.8223) (15.1606, 45.5312) knots 0 0 0 0 1 1 1 1
  spline S205 degree 3 poles (15.1606, 45.5312) (15.3723, 45.055) (15.6369, 44.5787) (15.875, 44.1025) knots 0 0 0 0 1 1 1 1
  spline S206 degree 3 poles (15.875, 44.1025) (15.9544, 43.9173) (16.1396, 43.8114) (16.3513, 43.8379) knots 0 0 0 0 1 1 1 1
  spline S207 degree 3 poles (16.3513, 43.8379) (16.801, 43.8643) (17.2508, 43.8908) (17.7006, 43.8908) knots 0 0 0 0 1 1 1 1
  spline S208 degree 3 poles (17.7006, 43.8908) (17.9652, 43.8908) (18.2298, 43.8379) (18.4679, 43.7321) knots 0 0 0 0 1 1 1 1
  spline S209 degree 3 poles (18.4679, 43.7321) (20.4788, 42.8589) (22.4896, 41.9594) (24.2888, 40.6894) knots 0 0 0 0 1 1 1 1
  spline S210 degree 3 poles (24.2888, 40.6894) (24.3417, 40.6364) (24.3946, 40.5835) (24.4475, 40.5042) knots 0 0 0 0 1 1 1 1
  spline S211 degree 3 poles (24.4475, 40.5042) (24.5004, 40.4777) (24.5533, 40.4777) (24.6063, 40.4512) knots 0 0 0 0 1 1 1 1
  spline S212 degree 2 poles (24.6063, 40.4512) (26.0615, 39.2077) (25.056, 36.9587) knots 0 0 0 1 1 1
  spline S213 degree 3 poles (25.056, 36.9587) (24.7385, 36.2973) (24.474, 35.5564) (24.0506, 34.9479) knots 0 0 0 0 1 1 1 1
  spline S214 degree 3 poles (24.0506, 34.9479) (23.1775, 33.7044) (22.86, 32.3285) (22.7277, 30.8469) knots 0 0 0 0 1 1 1 1
  spline S215 degree 3 poles (22.7277, 30.8469) (22.7013, 30.5029) (22.7013, 30.1325) (22.569, 29.8414) knots 0 0 0 0 1 1 1 1
  spline S216 degree 3 poles (22.569, 29.8414) (22.0133, 28.8096) (22.3044, 27.8306) (22.6748, 26.8517) knots 0 0 0 0 1 1 1 1
  spline S217 degree 3 poles (22.6748, 26.8517) (23.2304, 25.3964) (24.13, 24.2852) (25.3471, 23.3327) knots 0 0 0 0 1 1 1 1
  spline S218 degree 3 poles (25.3471, 23.3327) (26.0085, 22.83) (26.4583, 22.0627) (26.9875, 21.4012) knots 0 0 0 0 1 1 1 1
  spline S219 degree 3 poles (26.9875, 21.4012) (27.4108, 20.8456) (27.8077, 20.29) (28.1781, 19.7079) knots 0 0 0 0 1 1 1 1
  spline S220 degree 3 poles (28.1781, 19.7079) (28.2046, 19.655) (28.231, 19.6021) (28.2575, 19.5492) knots 0 0 0 0 1 1 1 1
  line L5 (28.2575, 19.5492) -> (28.866, 19.0994)
  spline S221 degree 3 poles (28.866, 19.0994) (29.5804, 19.1258) (30.2948, 19.1787) (30.9298, 18.6496) knots 0 0 0 0 1 1 1 1
  spline S222 degree 3 poles (30.9298, 18.6496) (32.1469, 17.6442) (32.3585, 16.2154) (31.459, 14.919) knots 0 0 0 0 1 1 1 1
  spline S223 degree 3 poles (31.459, 14.919) (31.0092, 14.2575) (30.5065, 13.596) (30.0831, 12.9346) knots 0 0 0 0 1 1 1 1
  spline S224 degree 3 poles (30.0831, 12.9346) (29.8979, 12.6435) (29.8185, 12.2996) (29.6863, 12.0085) knots 0 0 0 0 1 1 1 1
  spline S225 degree 3 poles (29.6863, 12.0085) (29.6863, 11.9556) (29.6863, 11.9027) (29.6863, 11.8498) knots 0 0 0 0 1 1 1 1
  spline S226 degree 3 poles (29.6863, 11.8498) (29.6598, 10.474) (29.6863, 9.0717) (29.6069, 7.6958) knots 0 0 0 0 1 1 1 1
  spline S227 degree 3 poles (29.6069, 7.6958) (29.554, 7.0079) (29.2894, 6.32) (29.1571, 5.6321) knots 0 0 0 0 1 1 1 1
  spline S228 degree 3 poles (29.1571, 5.6321) (29.1042, 5.4204) (29.0777, 5.1558) (29.1835, 4.9971) knots 0 0 0 0 1 1 1 1
  spline S229 degree 3 poles (29.1835, 4.9971) (29.6863, 4.124) (30.2154, 3.2508) (31.1415, 2.7481) knots 0 0 0 0 1 1 1 1
  spline S230 degree 3 poles (31.1415, 2.7481) (31.3531, 2.6423) (31.6442, 2.6423) (31.9088, 2.5894) knots 0 0 0 0 1 1 1 1
  spline S231 degree 3 poles (31.9088, 2.5894) (32.094, 2.5365) (32.2792, 2.4835) (32.4379, 2.4306) knots 0 0 0 0 1 1 1 1
  spline S232 degree 3 poles (32.4379, 2.4306) (32.5438, 2.4042) (32.6496, 2.4042) (32.7554, 2.4306) knots 0 0 0 0 1 1 1 1
  spline S233 degree 3 poles (32.7554, 2.4306) (33.8931, 2.854) (35.0573, 3.2773) (36.195, 3.7006) knots 0 0 0 0 1 1 1 1
  spline S234 degree 3 poles (36.195, 3.7006) (36.2744, 3.7271) (36.3538, 3.8594) (36.4067, 3.9388) knots 0 0 0 0 1 1 1 1
  spline S235 degree 3 poles (36.4067, 3.9388) (36.5125, 4.0975) (36.5654, 4.3886) (36.6977, 4.415) knots 0 0 0 0 1 1 1 1
  spline S236 degree 3 poles (36.6977, 4.415) (37.3327, 4.5738) (37.9942, 4.6796) (38.6556, 4.759) knots 0 0 0 0 1 1 1 1
  spline S237 degree 3 poles (38.6556, 4.759) (38.9202, 4.7854) (39.2113, 4.8119) (39.4758, 4.8119) knots 0 0 0 0 1 1 1 1
  spline S238 degree 3 poles (39.4758, 4.8119) (39.7404, 4.8119) (39.9521, 4.9971) (39.9785, 5.2352) knots 0 0 0 0 1 1 1 1
  spline S239 degree 3 poles (39.9785, 5.2352) (39.9785, 5.2881) (40.005, 5.3411) (40.005, 5.394) knots 0 0 0 0 1 1 1 1
  spline S240 degree 3 poles (39.9785, 5.394) (40.0844, 7.0608) (40.005, 8.7277) (41.1427, 10.0771) knots 0 0 0 0 1 1 1 1
  spline S241 degree 3 poles (41.1427, 10.0771) (41.275, 10.2358) (41.5396, 10.3417) (41.7513, 10.421) knots 0 0 0 0 1 1 1 1
  spline S242 degree 3 poles (41.7513, 10.421) (43.7621, 11.1354) (45.7729, 11.9292) (47.4133, 13.305) knots 0 0 0 0 1 1 1 1
  spline S243 degree 3 poles (47.4133, 13.305) (48.2335, 13.9929) (48.7892, 14.9983) (49.53, 15.7921) knots 0 0 0 0 1 1 1 1
  spline S244 degree 3 poles (49.53, 15.7921) (50.4031, 16.7446) (50.5883, 17.9088) (50.6413, 19.0994) knots 0 0 0 0 1 1 1 1
  spline S245 degree 3 poles (50.6413, 19.0994) (50.7471, 21.0308) (50.8529, 22.9358) (50.8794, 24.8673) knots 0 0 0 0 1 1 1 1
  spline S246 degree 3 poles (50.8794, 24.8673) (50.9058, 25.714) (50.7206, 26.5606) (50.6677, 27.4073) knots 0 0 0 0 1 1 1 1
  spline S247 degree 3 poles (50.6677, 27.4073) (50.6148, 28.1481) (51.435, 29.1271) (52.1494, 29.2858) knots 0 0 0 0 1 1 1 1
  spline S248 degree 3 poles (52.1494, 29.2858) (52.9696, 29.4446) (53.7898, 29.6033) (54.5835, 29.815) knots 0 0 0 0 1 1 1 1
  spline S249 degree 3 poles (54.5835, 29.815) (54.9804, 29.9208) (55.3773, 30.106) (55.7477, 30.3177) knots 0 0 0 0 1 1 1 1
  spline S250 degree 3 poles (55.7477, 30.3177) (56.7002, 30.8204) (58.0496, 30.6617) (58.8169, 29.9473) knots 0 0 0 0 1 1 1 1
  spline S251 degree 3 poles (58.8169, 29.9473) (59.2402, 29.5504) (59.7165, 29.2594) (59.7165, 28.4921) knots 0 0 0 0 1 1 1 1
  spline S252 degree 3 poles (59.7165, 28.4921) (59.7165, 28.1481) (60.3515, 27.7777) (60.7219, 27.4602) knots 0 0 0 0 1 1 1 1
  spline S253 degree 3 poles (60.7219, 27.4602) (61.1717, 27.0898) (61.6479, 26.7458) (62.0977, 26.3754) knots 0 0 0 0 1 1 1 1
  spline S254 degree 3 poles (62.0977, 26.3754) (62.3623, 26.1637) (62.5475, 25.8462) (62.6533, 25.5287) knots 0 0 0 0 1 1 1 1
  spline S255 degree 3 poles (62.6533, 25.5287) (63.1031, 24.2587) (64.0821, 23.3856) (65.114, 22.6183) knots 0 0 0 0 1 1 1 1
  spline S256 degree 3 poles (65.114, 22.6183) (65.9077, 22.0362) (66.8602, 22.0627) (67.7333, 22.4596) knots 0 0 0 0 1 1 1 1
  spline S257 degree 3 poles (67.7333, 22.4596) (69.3208, 23.1475) (70.8819, 23.8883) (72.4165, 24.6821) knots 0 0 0 0 1 1 1 1
  spline S258 degree 3 poles (72.4165, 24.6821) (72.9721, 24.9731) (73.4483, 25.4758) (73.951, 25.8727) knots 0 0 0 0 1 1 1 1
  spline S259 degree 3 poles (73.951, 25.8727) (74.2685, 26.1373) (74.586, 26.4548) (74.9035, 26.7194) knots 0 0 0 0 1 1 1 1
  spline S260 degree 3 poles (74.9035, 26.7194) (75.5915, 27.3015) (75.9354, 28.5979) (75.4592, 29.3388) knots 0 0 0 0 1 1 1 1
  spline S261 degree 3 poles (75.4592, 29.3388) (74.7183, 30.4765) (75.1681, 31.6671) (75.1417, 32.8313) knots 0 0 0 0 1 1 1 1
  spline S262 degree 3 poles (75.1417, 32.8313) (75.1417, 33.0429) (75.0358, 33.3075) (74.9035, 33.4927) knots 0 0 0 0 1 1 1 1
  spline S263 degree 3 poles (74.9035, 33.4927) (74.4273, 34.1542) (73.66, 34.2865) (72.9721, 34.604) knots 0 0 0 0 1 1 1 1
  spline S264 degree 3 poles (72.9721, 34.604) (71.7815, 35.1596) (70.7496, 36.0327) (69.8765, 37.0911) knots 0 0 0 0 1 1 1 1
  spline S265 degree 3 poles (69.8765, 37.0911) (68.4213, 38.8373) (67.5217, 40.9011) (66.3046, 42.8061) knots 0 0 0 0 1 1 1 1
  spline S266 degree 3 poles (66.3046, 42.8061) (66.0135, 43.2823) (65.696, 43.785) (65.2992, 44.1819) knots 0 0 0 0 1 1 1 1
  spline S267 degree 3 poles (65.2992, 44.1819) (64.6642, 44.8434) (64.77, 45.5842) (65.0346, 46.2986) knots 0 0 0 0 1 1 1 1
  spline S268 degree 3 poles (65.0346, 46.2986) (65.061, 46.3515) (65.061, 46.3779) (65.0875, 46.4309) knots 0 0 0 0 1 1 1 1
  spline S269 degree 3 poles (65.0875, 46.4309) (66.7015, 48.7063) (67.7863, 50.3996) (68.289, 51.1934) knots 0 0 0 0 1 1 1 1
  spline S270 degree 3 poles (68.289, 51.1934) (68.3948, 51.3256) (68.5006, 51.4579) (68.58, 51.6696) knots 0 0 0 0 1 1 1 1
  spline S271 degree 3 poles (68.58, 51.6696) (69.4531, 53.7333) (69.9558, 55.9029) (70.2204, 58.1254) knots 0 0 0 0 1 1 1 1
  spline S272 degree 3 poles (70.2204, 58.1254) (70.4321, 59.8452) (71.2523, 61.2211) (72.2577, 62.5704) knots 0 0 0 0 1 1 1 1
  spline S273 degree 3 poles (72.2577, 62.5704) (73.0515, 63.6552) (73.5277, 64.8988) (73.369, 66.3804) knots 0 0 0 0 1 1 1 1
  spline S274 degree 3 poles (73.369, 66.3804) (73.0515, 69.1321) (73.025, 71.8573) (74.5067, 74.3444) knots 0 0 0 0 1 1 1 1
  spline S275 degree 3 poles (74.5067, 74.3444) (75.565, 76.1171) (76.0677, 78.1279) (76.7292, 80.0594) knots 0 0 0 0 1 1 1 1
  spline S276 degree 3 poles (76.7292, 80.0594) (77.0202, 80.9061) (77.8404, 81.25) (78.396, 81.8586) knots 0 0 0 0 1 1 1 1
  spline S277 degree 3 poles (78.396, 81.8586) (78.449, 81.9115) (78.7665, 81.7527) (78.8723, 81.6469) knots 0 0 0 0 1 1 1 1
  spline S278 degree 3 poles (78.8723, 81.6469) (79.4015, 81.1177) (79.6396, 80.4563) (79.7719, 79.7684) knots 0 0 0 0 1 1 1 1
  spline S279 degree 3 poles (79.7719, 79.7684) (79.8248, 79.4509) (79.9306, 78.9482) (80.1423, 78.8688) knots 0 0 0 0 1 1 1 1
  spline S280 degree 3 poles (80.1423, 78.8688) (80.6715, 78.6571) (81.28, 78.5777) (81.8356, 78.6042) knots 0 0 0 0 1 1 1 1
  spline S281 degree 3 poles (81.8356, 78.6042) (82.2325, 78.6042) (82.6294, 78.8688) (83.0262, 79.0275) knots 0 0 0 0 1 1 1 1
  spline S282 degree 3 poles (83.0262, 79.0275) (83.185, 79.0804) (83.4231, 79.1598) (83.476, 79.3185) knots 0 0 0 0 1 1 1 1
  spline S283 degree 3 poles (83.476, 79.3185) (83.6083, 79.5831) (83.7671, 79.7948) (83.9787, 79.9536) knots 0 0 0 0 1 1 1 1
  spline S284 degree 3 poles (83.9787, 79.9536) (84.3227, 80.8796) (84.746, 82.0438) (85.1165, 82.9698) knots 0 0 0 0 1 1 1 1
  spline S285 degree 3 poles (85.1165, 82.9698) (85.0635, 83.4725) (85.0106, 84.0017) (84.9312, 84.5044) knots 0 0 0 0 1 1 1 1
  spline S286 degree 3 poles (84.9312, 84.5044) (84.746, 85.7744) (84.3756, 87.0179) (84.3492, 88.2615) knots 0 0 0 0 1 1 1 1
  spline S287 degree 3 poles (84.3492, 88.2615) (84.3227, 89.5844) (84.6402, 90.9073) (84.799, 92.2302) knots 0 0 0 0 1 1 1 1
  spline S288 degree 3 poles (84.799, 92.2302) (85.0106, 94.0294) (84.8519, 95.7756) (83.9523, 97.3896) knots 0 0 0 0 1 1 1 1
  spline S289 degree 3 poles (83.9523, 97.3896) (83.7142, 97.8394) (83.3967, 98.2627) (83.2379, 98.7125) knots 0 0 0 0 1 1 1 1
  spline S290 degree 3 poles (83.2379, 98.7125) (83.0792, 99.2152) (82.8939, 99.7973) (83.0262, 100.2736) knots 0 0 0 0 1 1 1 1
  spline S291 degree 3 poles (83.0262, 100.2736) (83.5289, 102.1256) (84.1904, 103.8984) (85.2752, 105.4859) knots 0 0 0 0 1 1 1 1
  spline S292 degree 3 poles (85.2752, 105.4859) (85.6985, 106.0944) (85.5133, 106.8088) (84.8783, 107.2057) knots 0 0 0 0 1 1 1 1
  spline S293 degree 3 poles (84.8783, 107.2057) (84.2698, 107.5761) (83.7671, 107.9994) (83.6348, 108.7667) knots 0 0 0 0 1 1 1 1
  spline S294 degree 3 poles (83.6348, 108.7667) (83.5819, 109.0048) (83.4231, 109.2165) (83.3702, 109.4546) knots 0 0 0 0 1 1 1 1
  spline S295 degree 3 poles (83.3702, 109.4546) (83.1056, 110.4865) (83.0262, 111.5184) (83.6612, 112.4709) knots 0 0 0 0 1 1 1 1
  spline S296 degree 3 poles (83.6612, 112.4709) (84.1904, 113.2381) (84.6137, 113.8996) (84.9577, 114.4552) knots 0 0 0 0 1 1 1 1
  spline S297 degree 3 poles (84.9577, 114.4552) (85.0635, 114.614) (85.1694, 114.7992) (85.2752, 114.9579) knots 0 0 0 0 1 1 1 1
  spline S298 degree 3 poles (85.2487, 114.9579) (86.2542, 116.6777) (86.4658, 117.4186) (86.4923, 117.7625) knots 0 0 0 0 1 1 1 1
  spline S299 degree 3 poles (86.4923, 117.7625) (86.4923, 117.8948) (86.5717, 118.0271) (86.7039, 118.1065) knots 0 0 0 0 1 1 1 1
  spline S300 degree 3 poles (86.7039, 118.1065) (86.7833, 118.1594) (86.8362, 118.2123) (86.8362, 118.2652) knots 0 0 0 0 1 1 1 1
  spline S301 degree 3 poles (86.8362, 118.2652) (86.9156, 118.5827) (86.9685, 118.9531) (86.9685, 119.2971) knots 0 0 0 0 1 1 1 1
  spline S302 degree 3 poles (86.9685, 119.2971) (87.0479, 120.1702) (86.7833, 120.4613) (85.9896, 120.8052) knots 0 0 0 0 1 1 1 1
  line L6 (85.2487, 114.9579) -> (85.2752, 114.9579)
  line L7 (39.9785, 5.394) -> (40.005, 5.394)
  line L8 (0, 0) -> (177.5497, 0) construction
  line L9 (177.5497, 0) -> (177.5497, 660) construction
  line L10 (177.5497, 660) -> (0, 660) construction
  line L11 (0, 660) -> (0, 0) construction
  spline S303 degree 3 poles (238.8826, 328.8719) (236.0895, 330.048) (233.2229, 329.2394) (230.5769, 328.8719) knots 0 0 0 0 1 1 1 1
  spline S304 degree 3 poles (230.5769, 328.8719) (228.0043, 328.5779) (226.1667, 329.1659) (224.4762, 330.7095) knots 0 0 0 0 1 1 1 1
  spline S305 degree 3 poles (224.4762, 330.7095) (224.0352, 331.1505) (223.5941, 331.8855) (223.5941, 332.4735) knots 0 0 0 0 1 1 1 1
  spline S306 degree 3 poles (223.5941, 332.4735) (223.6677, 334.1641) (223.8882, 335.8546) (224.0352, 337.5452) knots 0 0 0 0 1 1 1 1
  spline S307 degree 3 poles (224.0352, 337.5452) (224.0352, 337.6922) (224.1087, 337.8392) (224.1822, 337.9862) knots 0 0 0 0 1 1 1 1
  spline S308 degree 3 poles (224.1822, 337.9862) (224.9907, 339.6033) (225.5052, 341.5143) (221.9771, 347.762) knots 0 0 0 0 1 1 1 1
  spline S309 degree 2 poles (221.9771, 347.762) (221.9771, 347.8355) (221.9036, 347.909) knots 0 0 0 1 1 1
  spline S310 degree 3 poles (221.9036, 347.909) (221.6096, 348.6441) (221.3891, 349.3056) (221.0951, 350.0406) knots 0 0 0 0 1 1 1 1
  spline S311 degree 3 poles (221.0951, 350.0406) (219.625, 353.3482) (218.3755, 356.8028) (215.1414, 359.0814) knots 0 0 0 0 1 1 1 1
  spline S312 degree 3 poles (215.1414, 359.0814) (214.1124, 359.8164) (213.4508, 361.3599) (213.2303, 362.683) knots 0 0 0 0 1 1 1 1
  spline S313 degree 3 poles (213.2303, 362.683) (213.0098, 364.006) (213.5243, 365.4761) (213.7448, 366.7991) knots 0 0 0 0 1 1 1 1
  spline S314 degree 3 poles (213.7448, 366.7991) (214.1859, 369.7392) (214.3328, 372.7528) (215.8029, 375.4724) knots 0 0 0 0 1 1 1 1
  spline S315 degree 3 poles (215.8029, 375.4724) (216.9789, 377.6775) (216.3174, 380.4705) (214.1858, 381.8671) knots 0 0 0 0 1 1 1 1
  spline S316 degree 3 poles (214.1858, 381.8671) (212.9363, 382.7491) (212.3483, 383.8517) (212.3483, 385.4687) knots 0 0 0 0 1 1 1 1
  spline S317 degree 3 poles (212.3483, 385.4687) (212.3483, 386.7917) (211.8338, 387.7473) (210.4372, 388.3353) knots 0 0 0 0 1 1 1 1
  spline S318 degree 3 poles (210.4372, 388.3353) (208.5997, 389.0703) (207.1296, 390.3934) (206.1741, 392.2309) knots 0 0 0 0 1 1 1 1
  spline S319 degree 3 poles (206.1741, 392.2309) (205.8066, 392.9659) (204.9245, 393.4805) (204.1895, 393.9215) knots 0 0 0 0 1 1 1 1
  spline S320 degree 3 poles (204.1895, 393.9215) (200.9554, 395.906) (197.1333, 397.082) (195.5162, 400.9777) knots 0 0 0 0 1 1 1 1
  spline S321 degree 3 poles (195.5162, 400.9777) (194.8547, 402.5947) (194.1932, 404.2118) (193.6787, 405.8288) knots 0 0 0 0 1 1 1 1
  spline S322 degree 3 poles (193.6787, 405.8288) (192.2821, 409.8715) (193.0907, 412.5176) (196.4718, 415.1637) knots 0 0 0 0 1 1 1 1
  spline S323 degree 3 poles (196.4718, 415.1637) (198.2358, 416.5602) (200.1469, 417.8097) (200.4409, 420.3088) knots 0 0 0 0 1 1 1 1
  spline S324 degree 3 poles (200.4409, 420.3088) (200.7349, 422.9549) (202.1314, 425.16) (203.822, 427.218) knots 0 0 0 0 1 1 1 1
  spline S325 degree 3 poles (203.822, 427.218) (204.263, 427.806) (204.704, 428.3941) (204.998, 429.0556) knots 0 0 0 0 1 1 1 1
  spline S326 degree 3 poles (204.998, 429.0556) (205.2185, 429.4231) (205.4391, 429.9376) (205.292, 430.3051) knots 0 0 0 0 1 1 1 1
  spline S327 degree 3 poles (205.292, 430.3051) (204.41, 433.6863) (204.116, 437.2879) (200.8819, 439.6399) knots 0 0 0 0 1 1 1 1
  spline S328 degree 3 poles (200.8819, 439.6399) (198.1623, 441.6245) (196.0307, 444.1236) (195.1487, 447.5782) knots 0 0 0 0 1 1 1 1
  spline S329 degree 3 poles (195.1487, 447.5782) (195.0017, 448.0927) (194.8547, 448.6807) (194.9282, 449.1953) knots 0 0 0 0 1 1 1 1
  spline S330 degree 3 poles (194.9282, 449.1953) (195.5898, 453.5319) (197.9418, 456.9865) (201.6905, 459.1181) knots 0 0 0 0 1 1 1 1
  spline S331 degree 3 poles (201.6905, 459.1181) (205.2921, 461.1761) (209.1142, 462.8667) (212.7893, 464.8512) knots 0 0 0 0 1 1 1 1
  spline S332 degree 3 poles (212.7893, 464.8512) (213.5978, 465.2923) (214.4799, 465.8803) (214.8474, 466.6153) knots 0 0 0 0 1 1 1 1
  spline S333 degree 3 poles (214.8474, 466.6153) (215.7294, 468.6734) (217.126, 470.1434) (219.037, 471.3194) knots 0 0 0 0 1 1 1 1
  spline S334 degree 3 poles (219.037, 471.3194) (220.3601, 472.128) (222.1976, 472.9365) (222.7121, 474.186) knots 0 0 0 0 1 1 1 1
  spline S335 degree 3 poles (222.7121, 474.186) (223.6677, 476.3911) (224.6967, 478.8902) (222.6386, 481.2423) knots 0 0 0 0 1 1 1 1
  spline S336 degree 3 poles (222.6386, 481.2423) (220.5806, 483.5943) (222.0506, 485.1379) (224.5497, 485.7994) knots 0 0 0 0 1 1 1 1
  spline S337 degree 3 poles (224.5497, 485.7994) (226.4608, 486.3139) (228.4453, 486.5344) (230.2829, 487.1959) knots 0 0 0 0 1 1 1 1
  spline S338 degree 3 poles (230.2829, 487.1959) (231.6794, 487.7105) (233.37, 488.372) (233.958, 489.548) knots 0 0 0 0 1 1 1 1
  spline S339 degree 3 poles (233.958, 489.548) (235.2075, 491.9736) (236.0895, 494.6197) (236.6776, 497.3393) knots 0 0 0 0 1 1 1 1
  spline S340 degree 3 poles (236.6776, 497.3393) (236.9716, 498.8828) (236.7511, 500.7939) (236.0161, 502.1904) knots 0 0 0 0 1 1 1 1
  spline S341 degree 3 poles (236.0161, 502.1904) (235.281, 503.6605) (233.811, 504.763) (232.488, 505.792) knots 0 0 0 0 1 1 1 1
  spline S342 degree 3 poles (232.488, 505.792) (231.3119, 506.6741) (229.9154, 507.3356) (228.5188, 507.8501) knots 0 0 0 0 1 1 1 1
  spline S343 degree 3 poles (228.5188, 507.8501) (225.5052, 508.8791) (222.6387, 507.6296) (219.6986, 507.1151) knots 0 0 0 0 1 1 1 1
  spline S344 degree 3 poles (219.6986, 507.1151) (219.184, 507.0416) (218.5225, 506.8211) (218.0815, 507.0416) knots 0 0 0 0 1 1 1 1
  spline S345 degree 3 poles (218.0815, 507.0416) (217.273, 507.2621) (216.1704, 508.8056) (215.5089, 510.2022) knots 0 0 0 0 1 1 1 1
  spline S346 degree 3 poles (215.5089, 510.2022) (215.4354, 510.3492) (215.4354, 510.4227) (215.3619, 510.5697) knots 0 0 0 0 1 1 1 1
  spline S347 degree 3 poles (215.3619, 510.5697) (215.2149, 511.2312) (215.0679, 511.8192) (214.8474, 512.3337) knots 0 0 0 0 1 1 1 1
  spline S348 degree 3 poles (214.8474, 512.3337) (210.4372, 521.3745) (205.3656, 516.8909) (188.2395, 525.8582) knots 0 0 0 0 1 1 1 1
  spline S349 degree 3 poles (188.2395, 525.8582) (179.9337, 530.1948) (174.4211, 536.4425) (170.9665, 541.7347) knots 0 0 0 0 1 1 1 1
  spline S350 degree 3 poles (170.9665, 541.7347) (170.893, 541.8082) (170.893, 541.8817) (170.8195, 542.0287) knots 0 0 0 0 1 1 1 1
  spline S351 degree 3 poles (170.8195, 542.0287) (170.599, 542.6167) (170.3784, 543.1312) (170.1579, 543.7192) knots 0 0 0 0 1 1 1 1
  spline S352 degree 3 poles (170.1579, 543.7192) (169.9374, 544.1603) (169.7904, 544.6013) (169.4229, 544.7483) knots 0 0 0 0 1 1 1 1
  spline S353 degree 3 poles (169.4229, 544.7483) (169.2024, 544.8953) (168.9084, 545.0423) (168.7614, 545.3363) knots 0 0 0 0 1 1 1 1
  spline S354 degree 2 poles (168.7614, 545.3363) (166.7033, 549.1584) (165.8948, 551.8045) knots 0 0 0 1 1 1
  line L12 (165.8948, 551.8045) -> (165.8213, 552.319)
  spline S355 degree 3 poles (165.8213, 552.319) (165.6008, 554.6711) (166.9238, 556.2146) (168.6144, 557.7582) knots 0 0 0 0 1 1 1 1
  spline S356 degree 3 poles (168.6144, 557.7582) (168.9819, 558.1257) (169.1289, 559.0077) (169.0554, 559.6693) knots 0 0 0 0 1 1 1 1
  spline S357 degree 3 poles (169.0554, 559.6693) (168.9084, 561.0658) (168.0999, 561.9478) (166.7768, 562.5358) knots 0 0 0 0 1 1 1 1
  spline S358 degree 3 poles (166.7768, 562.5358) (166.5563, 562.6093) (166.3358, 562.7563) (166.1153, 562.9033) knots 0 0 0 0 1 1 1 1
  spline S359 degree 3 poles (166.1153, 562.9033) (165.3803, 563.3444) (165.2333, 564.3734) (165.8213, 565.0349) knots 0 0 0 0 1 1 1 1
  spline S360 degree 3 poles (165.8213, 565.0349) (166.5563, 565.8434) (167.2179, 566.2109) (168.2469, 566.2845) knots 0 0 0 0 1 1 1 1
  spline S361 degree 3 poles (168.2469, 566.2845) (169.1289, 566.358) (169.7169, 567.3135) (169.3494, 568.122) knots 0 0 0 0 1 1 1 1
  spline S362 degree 3 poles (169.3494, 568.122) (168.3939, 570.4006) (166.8504, 572.2381) (165.3068, 574.1492) knots 0 0 0 0 1 1 1 1
  spline S363 degree 3 poles (165.3068, 574.1492) (162.2197, 578.0448) (163.0282, 583.043) (167.2179, 585.2481) knots 0 0 0 0 1 1 1 1
  spline S364 degree 3 poles (167.2179, 585.2481) (168.3939, 585.8361) (169.7905, 585.9096) (171.2605, 586.0566) knots 0 0 0 0 1 1 1 1
  spline S365 degree 3 poles (171.2605, 586.0566) (172.069, 586.1301) (172.7305, 586.9386) (172.51, 587.7471) knots 0 0 0 0 1 1 1 1
  spline S366 degree 3 poles (172.51, 587.7471) (172.069, 589.2172) (171.481, 590.7607) (170.9665, 592.2308) knots 0 0 0 0 1 1 1 1
  spline S367 degree 3 poles (170.9665, 592.2308) (170.9665, 592.3043) (170.893, 592.3778) (170.893, 592.4513) knots 0 0 0 0 1 1 1 1
  spline S368 degree 3 poles (170.893, 592.4513) (169.9374, 594.0683) (169.7169, 595.8324) (170.0844, 597.7435) knots 0 0 0 0 1 1 1 1
  spline S369 degree 3 poles (170.0844, 597.7435) (170.452, 599.581) (170.452, 601.4186) (170.5255, 603.2561) knots 0 0 0 0 1 1 1 1
  spline S370 degree 3 poles (170.5255, 603.2561) (170.599, 604.7262) (169.7169, 605.5347) (168.4674, 605.9022) knots 0 0 0 0 1 1 1 1
  spline S371 degree 3 poles (168.4674, 605.9022) (167.8059, 606.1227) (167.0709, 606.2697) (166.3358, 606.4167) knots 0 0 0 0 1 1 1 1
  spline S372 degree 3 poles (166.3358, 606.4167) (163.3222, 607.0782) (161.4847, 609.8713) (161.6317, 612.8849) knots 0 0 0 0 1 1 1 1
  spline S373 degree 3 poles (161.6317, 612.8849) (161.7052, 614.208) (161.2642, 615.237) (160.1616, 616.1925) knots 0 0 0 0 1 1 1 1
  spline S374 degree 3 poles (160.1616, 616.1925) (157.8831, 618.3241) (157.3686, 621.1907) (158.6916, 624.0573) knots 0 0 0 0 1 1 1 1
  spline S375 degree 3 poles (158.6916, 624.0573) (158.8386, 624.3513) (158.9121, 624.7923) (158.7651, 624.9393) knots 0 0 0 0 1 1 1 1
  spline S376 degree 3 poles (158.7651, 624.9393) (157.8096, 626.3359) (157.2951, 628.2469) (155.09, 628.5409) knots 0 0 0 0 1 1 1 1
  spline S377 degree 3 poles (155.09, 628.5409) (124.954, 632.8776) (103.5648, 644.4175) (95.112, 650.4447) knots 0 0 0 0 1 1 1 1
  spline S378 degree 3 poles (95.112, 650.4447) (95.0385, 650.4447) (95.0385, 650.5182) (94.965, 650.5182) knots 0 0 0 0 1 1 1 1
  spline S379 degree 3 poles (94.965, 650.5182) (94.818, 650.6652) (94.671, 650.8122) (94.524, 650.9592) knots 0 0 0 0 1 1 1 1
  spline S380 degree 3 poles (94.524, 650.9592) (94.4505, 651.0327) (94.377, 651.1062) (94.3035, 651.1062) knots 0 0 0 0 1 1 1 1
  spline S381 degree 3 poles (94.3035, 651.1062) (94.1565, 651.1797) (94.0095, 651.3267) (93.789, 651.4002) knots 0 0 0 0 1 1 1 1